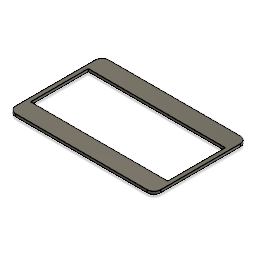
LCD Lid (Autodesk Fusion 360 design; units mm, degrees)
Autodesk Fusion 360 part; units mm, degrees
sketch "Sketch1" plane through (0, 0, 0) normal (0, 1, 0) x (1, 0, 0)
  line L0 (-52.5, 33.75) -> (52.5, 33.75)
  line L1 (52.5, 33.75) -> (52.5, -33.75)
  line L2 (52.5, -33.75) -> (-52.5, -33.75)
  line L3 (-52.5, -33.75) -> (-52.5, 33.75)
  line L4 (-52.5, 33.75) -> (52.5, -33.75) construction
  dimension "d115" = 105
  dimension "d116" = 67.5
  constraint horizontal L0
  constraint vertical L1
  constraint horizontal L2
  constraint vertical L3
  constraint midpoint origin L4
  measures "d115" distance of L0.start L0.end
  measures "d116" distance of L0.end L1.end
extrude "Extrude1" add sketch "Sketch1" along normal blind 2
fillet "Fillet1" radius 5 4 edges at (-52.5, 1, 33.75) (52.5, 1, 33.75) (52.5, 1, -33.75) (-52.5, 1, -33.75)
sketch "Sketch2" plane through (0, 2, 0) normal (0, 1, 0) x (-1, 0, 0)
  arc A0 (47.5, -33.75) -> (52.5, -28.75) centre (47.5, -28.75) ccw
  line L0 (52.5, -28.75) -> (52.5, 28.75)
  arc A1 (52.5, 28.75) -> (47.5, 33.75) centre (47.5, 28.75) ccw
  line L1 (47.5, 33.75) -> (-47.5, 33.75)
  arc A2 (-47.5, 33.75) -> (-52.5, 28.75) centre (-47.5, 28.75) ccw
  line L2 (-52.5, 28.75) -> (-52.5, -28.75)
  arc A3 (-52.5, -28.75) -> (-47.5, -33.75) centre (-47.5, -28.75) ccw
  line L3 (-47.5, -33.75) -> (47.5, -33.75)
  line L4 (49.5, -20.75) -> (-49.5, -20.75)
  line L5 (-49.5, -20.75) -> (-49.5, 20.75)
  line L6 (-49.5, 20.75) -> (49.5, 20.75)
  line L7 (49.5, 20.75) -> (49.5, -20.75)
  line L8 (49.5, -20.75) -> (-49.5, 20.75) construction
  dimension "d120" = 99
  dimension "d121" = 41.5
  constraint horizontal L4
  constraint vertical L5
  constraint horizontal L6
  constraint vertical L7
  constraint midpoint origin L8
  measures "d120" distance of L4.start L4.end
  measures "d121" distance of L4.start L6.end
extrude "Extrude2" cut sketch "Sketch2" against normal blind 2 contours L4 L5 L6 L7
sketch "Sketch3" plane through (0, 0, 0) normal (0, -1, 0) x (1, 0, 0)
  line L0 (49.5, 20.75) -> (49.5, -20.75)
  line L1 (49.5, -20.75) -> (-49.5, -20.75)
  line L2 (-49.5, -20.75) -> (-49.5, 20.75)
  line L3 (-49.5, 20.75) -> (49.5, 20.75)
  arc A0 (-52.5, -28.75) -> (-47.5, -33.75) centre (-47.5, -28.75) ccw
  line L4 (-47.5, -33.75) -> (47.5, -33.75)
  arc A1 (47.5, -33.75) -> (52.5, -28.75) centre (47.5, -28.75) ccw
  line L5 (52.5, -28.75) -> (52.5, 28.75)
  arc A2 (52.5, 28.75) -> (47.5, 33.75) centre (47.5, 28.75) ccw
  line L6 (47.5, 33.75) -> (-47.5, 33.75)
  arc A3 (-47.5, 33.75) -> (-52.5, 28.75) centre (-47.5, 28.75) ccw
  line L7 (-52.5, 28.75) -> (-52.5, -28.75)
  line L8 (-50.3, 28.75) -> (-50.3, -28.75)
  arc A4 (-50.3, -28.75) -> (-47.5, -31.55) centre (-47.5, -28.75) ccw
  line L9 (-47.5, -31.55) -> (47.5, -31.55)
  arc A5 (47.5, -31.55) -> (50.3, -28.75) centre (47.5, -28.75) ccw
  line L10 (50.3, -28.75) -> (50.3, 28.75)
  arc A6 (50.3, 28.75) -> (47.5, 31.55) centre (47.5, 28.75) ccw
  line L11 (47.5, 31.55) -> (-47.5, 31.55)
  arc A7 (-47.5, 31.55) -> (-50.3, 28.75) centre (-47.5, 28.75) ccw
  line L12 (-49.6448, 30.55) -> (49.6448, 30.55)
  line L13 (-49.6448, -30.55) -> (49.6448, -30.55)
  dimension "d124" = -2.2
  dimension "d125" = 1
  dimension "d126" = 1
  constraint coincident A7 L12.start
  constraint coincident A6 L12.end
  constraint horizontal L12
  constraint coincident A4 L13.start
  constraint coincident A5 L13.end
  constraint horizontal L13
  measures "d125" distance of L11 L12
  measures "d126" distance of L9 L13
extrude "Extrude3" add sketch "Sketch3" along normal blind 2 contours A6 L11 A7 L12 | A4 L9 A5 L13
